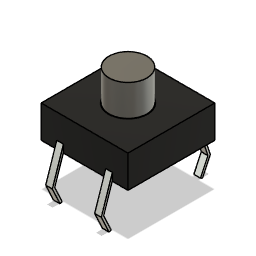
7.8mm button (Autodesk Fusion 360 design; units mm, degrees)
Autodesk Fusion 360 part; units mm, degrees
sketch "Sketch1" plane through (0, 0, 0) normal (0, 1, 0) x (1, 0, 0) in component "Base"
  line L0 (3.9, -3.9) -> (-3.9, -3.9)
  line L1 (-3.9, -3.9) -> (-3.9, 3.9)
  line L2 (-3.9, 3.9) -> (3.9, 3.9)
  line L3 (3.9, 3.9) -> (3.9, -3.9)
  line L4 (3.9, -3.9) -> (-3.9, 3.9) construction
  line L5 (-3.9, -3.9) -> (3.9, 3.9) construction
  dimension "d1" = 7.8
  dimension "d2" = 7.8
  constraint horizontal L0
  constraint perpendicular L0 L1
  constraint parallel L0 L2
  constraint parallel L1 L3
  constraint coincident L4 origin
  constraint coincident L5 origin
  measures "d1" distance of L1.end L2.end
  measures "d2" distance of L0.end L1.end
extrude "Extrude1" add sketch "Sketch1" along normal blind 2.9 makes body 1 in component "Base"
ref_plane "WorkPlane1" through (-3.9, 1.45, 0) normal (-1, 0, 0) x (0, 0, 1) in component "Base"
sketch "Sketch2" plane through (-3.9, 1.45, 0) normal (-1, 0, 0) x (0, 0, -1) in component "Base"
  line L0 (-3.9, 1.45) -> (3.9, 1.45) construction
  line L1 (-3.9, 1.45) -> (-4.9, 1.45) construction
  line L2 (-4.9, 1.45) -> (-4.9, 5.25) construction
  line L3 (3.9, 1.45) -> (4.9, 1.45) construction
  line L4 (4.9, 1.45) -> (4.9, 5.25) construction
  line L5 (-4.9, 5.25) -> (-4.2, 5.25) construction
  line L6 (4.9, 5.25) -> (4.2, 5.25) construction
  line L7 (4.9, 5.25) -> (4.9, 3.75) construction
  line L8 (-4.9, 5.25) -> (-4.9, 3.75) construction
  line L9 (-3.9, 1.45) -> (-3.9, 0.75) construction
  line L10 (3.9, 1.45) -> (3.9, -1.45) construction
  line L11 (-3.9, 0.75) -> (3.9, 0.75) construction
  line L12 (4.2, 5.25) -> (4.9, 3.75)
  line L13 (4.9, 3.75) -> (3.9, 0.75)
  line L14 (-4.2, 5.25) -> (-4.9, 3.75)
  line L15 (-4.9, 3.75) -> (-3.9, 0.75)
  line L16 (-4.0188, 5.1654) -> (-4.6851, 3.7376)
  line L17 (-4.6851, 3.7376) -> (-3.7103, 0.8132)
  line L18 (4.0188, 5.1654) -> (4.6851, 3.7376)
  line L19 (4.6851, 3.7376) -> (3.7103, 0.8132)
  line L20 (4.2, 5.25) -> (4.0188, 5.1654)
  line L21 (-4.0188, 5.1654) -> (-4.2, 5.25)
  line L22 (-3.9, 0.75) -> (-3.7103, 0.8132)
  line L23 (3.9, 0.75) -> (3.7103, 0.8132)
  point P0 (-3.9, 1.45)
  dimension "d6" = 1
  dimension "d7" = 3.8
  dimension "d8" = 1
  dimension "d9" = 3.8
  dimension "d10" = 0.7
  dimension "d11" = 0.7
  dimension "d12" = 1.5
  dimension "d13" = 1.5
  dimension "d14" = 0.7
  dimension "d15" = -0.2
  dimension "d16" = 0.2
  constraint coincident P0 L0.start
  constraint parallel L0 L1
  constraint perpendicular L0 L2
  constraint coincident L0.end L3.start
  constraint perpendicular L2 L3
  constraint perpendicular L0 L4
  constraint perpendicular L2 L5
  constraint perpendicular L2 L6
  constraint perpendicular L6 L7
  constraint perpendicular L5 L8
  constraint perpendicular L0 L9
  constraint coincident L10 L11.end
  constraint perpendicular L9 L11
  constraint perpendicular L14 L21
  measures "d6" distance of P0 L1.end
  measures "d7" distance of L1.end L2.end
  measures "d8" distance of L0.end L3.end
  measures "d9" distance of L3.end L4.end
  measures "d10" distance of L2.end L5.end
  measures "d11" distance of L4.end L6.end
  measures "d12" distance of L4.end L7.end
  measures "d13" distance of L2.end L8.end
  measures "d14" distance of P0 L9.end
extrude "Extrude2" add sketch "Sketch2" along normal blind -6.4 and the other way blind 5.8 separate body makes body 2 at (2.1, -1.3, -4.5667) makes body 3 at (2.1, -1.3, 4.5667) in component "Base"
extrude "Extrude3" add sketch "Sketch2" along normal blind -2 and the other way blind 1.4 separate body makes body 4 at (-2.3, -1.3, 4.5667) makes body 5 at (-2.3, -1.3, -4.5667) in component "Base"
combine "Combine1" operation add target body 1 tool bodies 4 3 2 5 in component "Base"
sketch "Sketch1 (2)" plane through (0, 2.9, 0) normal (0, 1, 0) x (-1, 0, 0) in component "Button"
  line L0 (-3.9, -3.9) -> (3.9, -3.9)
  line L1 (3.9, -3.9) -> (3.9, 3.9)
  line L2 (3.9, 3.9) -> (-3.9, 3.9)
  line L3 (-3.9, 3.9) -> (-3.9, -3.9)
  circle A0 centre (0, 0) radius 1.7
  dimension "d25" = 3.4
  constraint coincident A0.centre origin
  measures "d25" diameter of A0
extrude "Extrude1'" add sketch "Sketch1 (2)" along normal blind 2.8 separate body contours A0 makes body 6 in component "Button"
sketch "Sketch3" plane through (0, 2.9, 0) normal (0, 1, 0) x (-1, 0, 0) in component "Base"
  line L0 (-3.9, -3.9) -> (3.9, -3.9)
  line L1 (3.9, -3.9) -> (3.9, 3.9)
  line L2 (3.9, 3.9) -> (-3.9, 3.9)
  line L3 (-3.9, 3.9) -> (-3.9, -3.9)
  circle A0 centre (0, 0) radius 1.75
  dimension "d28" = 3.5
  constraint coincident A0.centre origin
  measures "d28" diameter of A0
extrude "Extrude4" cut sketch "Sketch3" against normal blind 1.6 contours A0 bodies 1 in component "Base"
component "Base" placed x (1, 0, 0) y (0, 1, 0) z (0, 0, 1) at (0, 0, 0)
component "Button" placed x (1, 0, 0) y (0, 1, 0) z (0, 0, 1) at (0, 0, 0)
equation "d17 = -7.80 mm + 1.4 mm"
equation "d19 = 6.4 mm - 0.6 mm"
